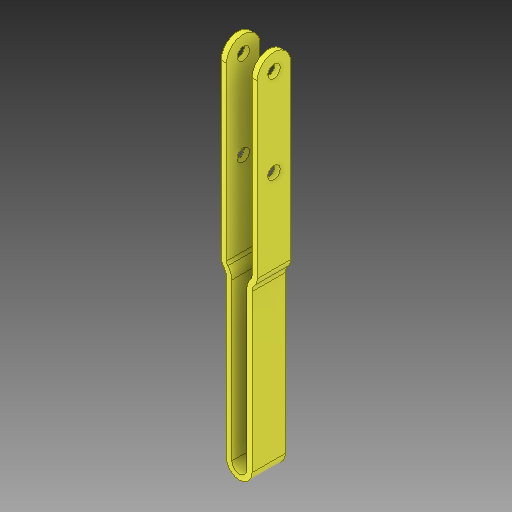
# Autodesk Inventor part: Part5
Saved by Autodesk Inventor 2019 (Build 230136000, 136)
## iProperties
Created: 2018-10-25
Part Number: Part5
Material: Iron, Gray
Document SubType Name: Sheet Metal
Designer: Isaac
Density: 7.15 g/cm^3
Flat Pattern Width: 1.6 cm
Flat Pattern Length: 35.8787 cm
Flat Pattern Area: 57.4058 cm^2
Sheet Metal Rule: Default_mm
Sheet Metal Width: 16.000 mm
Sheet Metal Length: 358.787 mm
Sheet Metal Area: 5740.584 mm^2
Appearance: Smooth - Yellow
Mass: 99.8681 g
Surface Area: 132.067 cm^2
Volume: 13.9676 cm^3
Author: Isaac
Autodesk Inventor part; units mm, degrees
ref_plane "YZ Plane" through (0, 0, 0) normal (1, 0, 0) x (0, 1, 0)
ref_plane "XZ Plane" through (0, 0, 0) normal (0, 1, 0) x (-1, 0, 0)
ref_plane "XY Plane" through (0, 0, 0) normal (0, 0, 1) x (1, 0, 0)
sketch "Sketch1" plane through (0, 0, 0) normal (0, 0, 1) x (1, 0, 0)
  line L0 (0, 104.6011) -> (0, -104.6011)
  line L1 (-8.6, 115.3268) -> (-8.6, 25.3268)
  arc A0 (-8.6, 25.3268) -> (-7.35, 22.0196) centre (-3.6, 25.3268) ccw
  arc A1 (-6.1, 18.7124) -> (-7.35, 22.0196) centre (-11.1, 18.7124) ccw
  line L2 (-6.1, 18.7124) -> (-6.1, -56.2876)
  arc A2 (-6.1, -56.2876) -> (0, -62.3876) centre (0, -56.2876) ccw
  arc A3 (-3.6, -56.2876) -> (0, -59.8876) centre (0, -56.2876) ccw
  line L3 (-3.6, -56.2876) -> (-3.6, 18.7124)
  arc A4 (-3.6, 18.7124) -> (-5.475, 23.6732) centre (-11.1, 18.7124) ccw
  arc A5 (-6.1, 25.3268) -> (-5.475, 23.6732) centre (-3.6, 25.3268) ccw
  line L4 (-6.1, 25.3268) -> (-6.1, 115.3268)
  line L5 (-8.6, 115.3268) -> (-6.1, 115.3268)
  line L6 (8.6, 115.3268) -> (8.6, 25.3268)
  arc A6 (7.35, 22.0196) -> (8.6, 25.3268) centre (3.6, 25.3268) ccw
  arc A7 (7.35, 22.0196) -> (6.1, 18.7124) centre (11.1, 18.7124) ccw
  line L7 (6.1, 18.7124) -> (6.1, -56.2876)
  arc A8 (0, -62.3876) -> (6.1, -56.2876) centre (0, -56.2876) ccw
  arc A9 (0, -59.8876) -> (3.6, -56.2876) centre (0, -56.2876) ccw
  line L8 (3.6, -56.2876) -> (3.6, 18.7124)
  arc A10 (5.475, 23.6732) -> (3.6, 18.7124) centre (11.1, 18.7124) ccw
  arc A11 (5.475, 23.6732) -> (6.1, 25.3268) centre (3.6, 25.3268) ccw
  line L9 (6.1, 25.3268) -> (6.1, 115.3268)
  line L10 (8.6, 115.3268) -> (6.1, 115.3268)
  point P0 (0, 0)
  point P1 (0, 0)
  dimension "d0" = 90
  dimension "d1" = 5
  dimension "d2" = 75
  dimension "d3" = 6.1
  dimension "d4" = 6.1
  dimension "d5" = 8.6
  dimension "d6" = 2.5
  constraints: 24 point on circle, 22 end point, 12 centre point, 12 symmetric about line, 4 tangent, 3 vertical, 2 coincident, 1 equal radius, 1 horizontal, 1 line through centre, 1 midpoint, 1 point on line, 10 other
  measures "d0" distance of L1.start L1.end
  measures "d1" radius of A0
  measures "d2" distance of L2.start L2.end
  measures "d3" radius of A2
  measures "d4" distance between parallel lines of L2 L0
  measures "d5" distance between parallel lines of L1 L0
  measures "d6" distance between parallel lines of L1 L4
extrude "Extrusion1" add sketch "Sketch1" along normal mid plane 16
hole "Hole1" at (8.6, 107.3268, 0) direction (-1, 0, 0) diameter 6 depth 30 tip angle 118
hole "Hole2" at (8.6, 65.3268, 0) direction (-1, 0, 0) diameter 6 depth 30 tip angle 118
fillet "Fillet1" radius 8 4 edges at (7.35, 115.3268, -8) (7.35, 115.3268, 8) (-7.35, 115.3268, 8) (-7.35, 115.3268, -8)
equation "\"BendRadius\" = Thickness"
equation "\"BendReliefWidth\" = Thickness"
equation "\"BendReliefDepth\" = 0.5 * Thickness"
equation "\"MinimumRemnant\" = 2 * Thickness"
equation "\"TransitionRadius\" = BendRadius"
equation "\"JacobiRadiusSize\" = BendRadius"
equation "\"GapSize\" = Thickness"
equation "\"Thickness\" = 2.5"
body "Solid1"
